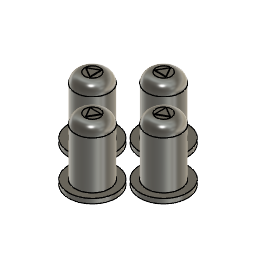
Buttons (Autodesk Fusion 360 archive; units mm, degrees)
design "D-pad"
part number: 2025-12-04-00-47-35-173
Autodesk Fusion 360 part; units mm, degrees
sketch "Sketch7" plane through (0, 0, 0) normal (0, 0, 1) x (1, 0, 0)
  circle A0 through (227.5, 10.5, -5) (220, 14.8301, -5) (220, 6.1699, -5)
  circle A1 through (226.075, 10.5, -5) (220.7125, 13.596, -5) (220.7125, 7.404, -5)
  circle A2 through (224.25, 10.5, -5) (221.625, 12.0155, -5) (221.625, 8.9845, -5)
  circle A3 through (220, 3, -5) (212.5, 7.3301, -5) (212.5, -1.3301, -5)
  circle A4 through (218.575, 3, -5) (213.2125, 6.096, -5) (213.2125, -0.096, -5)
  circle A5 through (216.75, 3, -5) (214.125, 4.5155, -5) (214.125, 1.4845, -5)
  line L0 (218, 6, -5) -> (212, 0, -5) construction
  line L1 (218, 6, -5) -> (212, 6, -5) construction
  circle A6 through (212.5, 10.5, -5) (205, 14.8301, -5) (205, 6.1699, -5)
  circle A7 through (211.075, 10.5, -5) (205.7125, 13.596, -5) (205.7125, 7.404, -5)
  circle A8 through (209.25, 10.5, -5) (206.625, 12.0155, -5) (206.625, 8.9845, -5)
  circle A9 through (218.575, 18, -5) (213.2125, 21.096, -5) (213.2125, 14.904, -5)
  circle A10 through (220, 18, -5) (212.5, 22.3301, -5) (212.5, 13.6699, -5)
  circle A11 through (216.75, 18, -5) (214.125, 19.5155, -5) (214.125, 16.4845, -5)
  point P0 (215, 3)
  dimension "d709" = 7.15
  dimension "d710" = 3.5
  dimension "d711" = 10
  dimension "d712" = 3.5
  dimension "d713" = 7.15
  dimension "d714" = 10
  dimension "d715" = 3.5
  dimension "d716" = 7.15
  dimension "d717" = 10
  dimension "d718" = 7.15
  dimension "d719" = 3.5
  dimension "d720" = 10
  dimension "d721" = 6
extrude "Extrude3" add sketch "Sketch7" along normal blind 13 contours A1 | A2 | A4 | A5 | A7 | A8 | A9 | A11 in plane through (0, 0, -5) normal (0, 0, 1) makes body 1 at (216.1386, 21.3888, 3.6667) makes body 2 at (206.3614, 7.1112, 3.6667) makes body 3 at (221.3614, 7.1112, 3.6667) makes body 4 at (216.1386, 6.3888, 3.6667)
extrude "Extrude4" add sketch "Sketch7" along normal blind 1 contours A0 | A3 | A6 | A10 in plane through (0, 0, -5) normal (0, 0, 1) bodies 1 2 3 4
extrude "Extrude5" cut sketch "Sketch7" along normal blind 6 contours A2 | A5 | A8 | A11 in plane through (0, 0, -5) normal (0, 0, 1) bodies 1 2 3 4
fillet "Fillet2" radius 2 4 faces at (216.1387, 17.6488, 8) (208.6387, 10.1488, 8) (223.6387, 10.1488, 8) (216.1387, 2.6488, 8) on bodies 1 2 3 4
sketch "Sketch9" plane through (0, 0, 8) normal (0, 0, 1) x (-1, 0, 0)
  circle A0 centre (-222.5, -10.5) radius 1.575
  line L0 (-226.5, -6.5) -> (-218.5, -6.5) construction
  line L1 (-218.5, -6.5) -> (-218.5, -14.5) construction
  line L2 (-218.5, -14.5) -> (-226.5, -14.5) construction
  line L3 (-226.5, -14.5) -> (-226.5, -6.5) construction
  line L4 (-226.5, -6.5) -> (-218.5, -14.5) construction
  line L5 (-218.5, -6.5) -> (-226.5, -14.5) construction
  line L6 (-203.5, -14.5) -> (-211.5, -14.5) construction
  line L7 (-211.5, -14.5) -> (-211.5, -6.5) construction
  line L8 (-211.5, -6.5) -> (-203.5, -6.5) construction
  line L9 (-203.5, -6.5) -> (-203.5, -14.5) construction
  line L10 (-203.5, -14.5) -> (-211.5, -6.5) construction
  line L11 (-211.5, -14.5) -> (-203.5, -6.5) construction
  line L12 (-207.5, -10.5) -> (-222.5, -10.5) construction
  line L13 (-219, 1) -> (-211, 1) construction
  line L14 (-211, 1) -> (-211, -7) construction
  line L15 (-211, -7) -> (-219, -7) construction
  line L16 (-219, -7) -> (-219, 1) construction
  line L17 (-219, 1) -> (-211, -7) construction
  line L18 (-211, 1) -> (-219, -7) construction
  line L19 (-219, -14) -> (-211, -14) construction
  line L20 (-211, -14) -> (-211, -22) construction
  line L21 (-211, -22) -> (-219, -22) construction
  line L22 (-219, -22) -> (-219, -14) construction
  line L23 (-219, -14) -> (-211, -22) construction
  line L24 (-211, -14) -> (-219, -22) construction
  line L25 (-215, -18) -> (-215, -3) construction
  line L26 (-206, -9) -> (-209, -9) construction
  line L27 (-209, -9) -> (-209, -12) construction
  line L28 (-209, -12) -> (-206, -12) construction
  line L29 (-206, -12) -> (-206, -9) construction
  line L30 (-206, -9) -> (-209, -12) construction
  line L31 (-209, -9) -> (-206, -12) construction
  line L32 (-223, -10.5) -> (-222, -10.5) construction
  line L33 (-221.796, -9.2899) -> (-223.9, -10.4954)
  line L34 (-223.9, -10.4954) -> (-221.804, -11.7147)
  line L35 (-221.804, -11.7147) -> (-221.796, -9.2899)
  line L36 (-208.2, -11.7124) -> (-206.1, -10.5)
  line L37 (-206.1, -10.5) -> (-208.2, -9.2876)
  line L38 (-208.2, -9.2876) -> (-208.2, -11.7124)
  line L39 (-221, -9) -> (-224, -9) construction
  line L40 (-224, -9) -> (-224, -12) construction
  line L41 (-224, -12) -> (-221, -12) construction
  line L42 (-221, -12) -> (-221, -9) construction
  line L43 (-221, -9) -> (-224, -12) construction
  line L44 (-224, -9) -> (-221, -12) construction
  line L45 (-216.2124, -17.3) -> (-215, -19.4)
  line L46 (-215, -19.4) -> (-213.7876, -17.3)
  line L47 (-213.7876, -17.3) -> (-216.2124, -17.3)
  line L48 (-213.7876, -3.7) -> (-215, -1.6)
  line L49 (-215, -1.6) -> (-216.2124, -3.7)
  line L50 (-216.2124, -3.7) -> (-213.7876, -3.7)
  point P0 (-222.5, -10.5)
  point P1 (-215, -3)
  point P2 (-215, -18)
  point P3 (-207.5, -10.5)
  point P4 (-222.5, -10.5)
  point P5 (-207.5, -10.5)
  point P6 (-222.5, -10.5)
  point P7 (-215, -18)
  point P8 (-215, -3)
  dimension "d731" = 8
  dimension "d732" = 8
  dimension "d735" = 8
  dimension "d736" = 8
  dimension "d737" = 8
  dimension "d738" = 8
  dimension "d739" = 8
  dimension "d740" = 8
  constraint horizontal L0
  constraint perpendicular L0 L1
  constraint parallel L0 L2
  constraint parallel L1 L3
  constraint coincident L4 P4
  constraint coincident L5 P4
  constraint coincident P4 P0
  constraint horizontal L6
  constraint vertical L7
  constraint horizontal L8
  constraint vertical L9
  constraint perpendicular L10 L11
  constraint midpoint L11 P5
  constraint horizontal L13
  constraint perpendicular L13 L14
  constraint parallel L13 L15
  constraint parallel L14 L16
  constraint coincident L17 P8
  constraint coincident L18 P8
  constraint horizontal L19
  constraint perpendicular L19 L20
  constraint parallel L19 L21
  constraint parallel L20 L22
  constraint coincident L23 P7
  constraint coincident L24 P7
  constraint coincident P7 P2
  constraint coincident P8 P1
  constraint perpendicular L15 L25
  constraint horizontal L26
  constraint perpendicular L26 L27
  constraint parallel L26 L28
  constraint parallel L27 L29
  constraint coincident L30 P5
  constraint coincident L31 P5
  constraint coincident L11 L26.start
  constraint coincident P5 P3
  constraint coincident L12 L32.end
  constraint horizontal L39
  constraint perpendicular L39 L40
  constraint parallel L39 L41
  constraint parallel L40 L42
  constraint coincident L43 P6
  constraint coincident L44 P6
  constraint coincident L5 L39.start
  constraint coincident P6 P4
  measures "d731" distance of L1.end L2.end
  measures "d732" distance of L0.end L1.end
  measures "d735" distance of L14.end L15.end
  measures "d736" distance of L13.end L14.end
  measures "d737" distance of L20.end L21.end
  measures "d738" distance of L19.end L20.end
  measures "d739" distance of L6.start L6.end
  measures "d740" distance of L6.start L8.end
extrude "Extrude7" add sketch "Sketch9" along normal blind 0.1 contours L33 L34 L35 | L36 L37 L38 | L45 L46 L47 | L48 L49 L50 bodies 1 2 3 4
fillet "Fillet3" radius 0.025 4 faces at (215, 18, 8.1) (207.5, 10.5, 8.1) (222.5, 10.5, 8.1) (215, 3, 8.1) on bodies 1 2 3 4
sketch "sketch 1269" plane through (314.9238, 31, 1.0977) normal (0, 0, 1) x (-1, 0, 0)
  circle A0 centre (99.9671, 27.0078) radius 3.6
  circle A1 centre (99.9671, 27.0078) radius 3.6
  circle A2 centre (107.4671, 19.5078) radius 3.6
  circle A3 centre (107.4671, 19.5078) radius 3.6
  circle A4 centre (99.9671, -15.4922) radius 10.5
  circle A5 centre (99.9671, -15.4922) radius 10.5
  circle A6 centre (99.9671, 12.0078) radius 3.6
  circle A7 centre (99.9671, 12.0078) radius 3.6
  circle A8 centre (92.4675, 19.584) radius 3.5995
extrude "Extrude8" cut sketch "sketch 1269" against normal blind 3 bodies 1 2 3 4
delete_face "DeleteFace1" 1 faces at (212.095, 3.0837, -1.9023) on bodies 4
delete_face "DeleteFace2" 1 faces at (204.595, 10.5837, -1.9023) on bodies 2
delete_face "DeleteFace3" 1 faces at (212.095, 18.0837, -1.9023) on bodies 1
delete_face "DeleteFace4" 1 faces at (219.5655, 10.889, -1.9023) on bodies 3

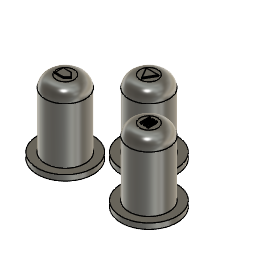
design "Menu"
part number: 2025-12-04-00-47-35-173
Autodesk Fusion 360 part; units mm, degrees
sketch "Sketch7" plane through (0, 0, 0) normal (0, 0, 1) x (1, 0, 0)
  circle A0 through (227.5, 10.5, -5) (220, 14.8301, -5) (220, 6.1699, -5)
  circle A1 through (226.075, 10.5, -5) (220.7125, 13.596, -5) (220.7125, 7.404, -5)
  circle A2 through (224.25, 10.5, -5) (221.625, 12.0155, -5) (221.625, 8.9845, -5)
  circle A3 through (220, 3, -5) (212.5, 7.3301, -5) (212.5, -1.3301, -5)
  circle A4 through (218.575, 3, -5) (213.2125, 6.096, -5) (213.2125, -0.096, -5)
  circle A5 through (216.75, 3, -5) (214.125, 4.5155, -5) (214.125, 1.4845, -5)
  line L0 (218, 6, -5) -> (212, 0, -5) construction
  line L1 (218, 6, -5) -> (212, 6, -5) construction
  circle A6 through (212.5, 10.5, -5) (205, 14.8301, -5) (205, 6.1699, -5)
  circle A7 through (211.075, 10.5, -5) (205.7125, 13.596, -5) (205.7125, 7.404, -5)
  circle A8 through (209.25, 10.5, -5) (206.625, 12.0155, -5) (206.625, 8.9845, -5)
  circle A9 through (218.575, 18, -5) (213.2125, 21.096, -5) (213.2125, 14.904, -5)
  circle A10 through (220, 18, -5) (212.5, 22.3301, -5) (212.5, 13.6699, -5)
  circle A11 through (216.75, 18, -5) (214.125, 19.5155, -5) (214.125, 16.4845, -5)
  point P0 (215, 3)
  dimension "d709" = 7.15
  dimension "d710" = 3.5
  dimension "d711" = 10
  dimension "d712" = 3.5
  dimension "d713" = 7.15
  dimension "d714" = 10
  dimension "d715" = 3.5
  dimension "d716" = 7.15
  dimension "d717" = 10
  dimension "d718" = 7.15
  dimension "d719" = 3.5
  dimension "d720" = 10
  dimension "d721" = 6
extrude "Extrude3" add sketch "Sketch7" along normal blind 13 contours A1 | A2 | A4 | A5 | A7 | A8 | A9 | A11 in plane through (0, 0, -5) normal (0, 0, 1) makes body 1 at (216.1386, 21.3888, 3.6667) makes body 2 at (206.3614, 7.1112, 3.6667) makes body 3 at (221.3614, 7.1112, 3.6667) makes body 4 at (216.1386, 6.3888, 3.6667)
extrude "Extrude4" add sketch "Sketch7" along normal blind 1 contours A0 | A3 | A6 | A10 in plane through (0, 0, -5) normal (0, 0, 1) bodies 1 2 3 4
extrude "Extrude5" cut sketch "Sketch7" along normal blind 6 contours A2 | A5 | A8 | A11 in plane through (0, 0, -5) normal (0, 0, 1) bodies 1 2 3 4
fillet "Fillet2" radius 2 4 faces at (216.1387, 17.6488, 8) (208.6387, 10.1488, 8) (223.6387, 10.1488, 8) (216.1387, 2.6488, 8) on bodies 1 2 3 4
sketch "Sketch9" plane through (0, 0, 8) normal (0, 0, 1) x (-1, 0, 0)
  circle A0 centre (-222.5, -10.5) radius 1.575
  line L0 (-226.5, -6.5) -> (-218.5, -6.5) construction
  line L1 (-218.5, -6.5) -> (-218.5, -14.5) construction
  line L2 (-218.5, -14.5) -> (-226.5, -14.5) construction
  line L3 (-226.5, -14.5) -> (-226.5, -6.5) construction
  line L4 (-226.5, -6.5) -> (-218.5, -14.5) construction
  line L5 (-218.5, -6.5) -> (-226.5, -14.5) construction
  line L6 (-203.5, -14.5) -> (-211.5, -14.5) construction
  line L7 (-211.5, -14.5) -> (-211.5, -6.5) construction
  line L8 (-211.5, -6.5) -> (-203.5, -6.5) construction
  line L9 (-203.5, -6.5) -> (-203.5, -14.5) construction
  line L10 (-203.5, -14.5) -> (-211.5, -6.5) construction
  line L11 (-211.5, -14.5) -> (-203.5, -6.5) construction
  line L12 (-207.5, -10.5) -> (-222.5, -10.5) construction
  line L13 (-219, 1) -> (-211, 1) construction
  line L14 (-211, 1) -> (-211, -7) construction
  line L15 (-211, -7) -> (-219, -7) construction
  line L16 (-219, -7) -> (-219, 1) construction
  line L17 (-219, 1) -> (-211, -7) construction
  line L18 (-211, 1) -> (-219, -7) construction
  line L19 (-219, -14) -> (-211, -14) construction
  line L20 (-211, -14) -> (-211, -22) construction
  line L21 (-211, -22) -> (-219, -22) construction
  line L22 (-219, -22) -> (-219, -14) construction
  line L23 (-219, -14) -> (-211, -22) construction
  line L24 (-211, -14) -> (-219, -22) construction
  line L25 (-215, -18) -> (-215, -3) construction
  line L26 (-206, -9) -> (-209, -9) construction
  line L27 (-209, -9) -> (-209, -12) construction
  line L28 (-209, -12) -> (-206, -12) construction
  line L29 (-206, -12) -> (-206, -9) construction
  line L30 (-206, -9) -> (-209, -12) construction
  line L31 (-209, -9) -> (-206, -12) construction
  line L32 (-223, -10.5) -> (-222, -10.5) construction
  line L33 (-221.796, -9.2899) -> (-223.9, -10.4954)
  line L34 (-223.9, -10.4954) -> (-221.804, -11.7147)
  line L35 (-221.804, -11.7147) -> (-221.796, -9.2899)
  line L36 (-208.2, -11.7124) -> (-206.1, -10.5)
  line L37 (-206.1, -10.5) -> (-208.2, -9.2876)
  line L38 (-208.2, -9.2876) -> (-208.2, -11.7124)
  line L39 (-221, -9) -> (-224, -9) construction
  line L40 (-224, -9) -> (-224, -12) construction
  line L41 (-224, -12) -> (-221, -12) construction
  line L42 (-221, -12) -> (-221, -9) construction
  line L43 (-221, -9) -> (-224, -12) construction
  line L44 (-224, -9) -> (-221, -12) construction
  line L45 (-216.2124, -17.3) -> (-215, -19.4)
  line L46 (-215, -19.4) -> (-213.7876, -17.3)
  line L47 (-213.7876, -17.3) -> (-216.2124, -17.3)
  line L48 (-213.7876, -3.7) -> (-215, -1.6)
  line L49 (-215, -1.6) -> (-216.2124, -3.7)
  line L50 (-216.2124, -3.7) -> (-213.7876, -3.7)
  point P0 (-222.5, -10.5)
  point P1 (-215, -3)
  point P2 (-215, -18)
  point P3 (-207.5, -10.5)
  point P4 (-222.5, -10.5)
  point P5 (-207.5, -10.5)
  point P6 (-222.5, -10.5)
  point P7 (-215, -18)
  point P8 (-215, -3)
  dimension "d731" = 8
  dimension "d732" = 8
  dimension "d735" = 8
  dimension "d736" = 8
  dimension "d737" = 8
  dimension "d738" = 8
  dimension "d739" = 8
  dimension "d740" = 8
  constraint horizontal L0
  constraint perpendicular L0 L1
  constraint parallel L0 L2
  constraint parallel L1 L3
  constraint coincident L4 P4
  constraint coincident L5 P4
  constraint coincident P4 P0
  constraint horizontal L6
  constraint vertical L7
  constraint horizontal L8
  constraint vertical L9
  constraint perpendicular L10 L11
  constraint midpoint L11 P5
  constraint horizontal L13
  constraint perpendicular L13 L14
  constraint parallel L13 L15
  constraint parallel L14 L16
  constraint coincident L17 P8
  constraint coincident L18 P8
  constraint horizontal L19
  constraint perpendicular L19 L20
  constraint parallel L19 L21
  constraint parallel L20 L22
  constraint coincident L23 P7
  constraint coincident L24 P7
  constraint coincident P7 P2
  constraint coincident P8 P1
  constraint perpendicular L15 L25
  constraint horizontal L26
  constraint perpendicular L26 L27
  constraint parallel L26 L28
  constraint parallel L27 L29
  constraint coincident L30 P5
  constraint coincident L31 P5
  constraint coincident L11 L26.start
  constraint coincident P5 P3
  constraint coincident L12 L32.end
  constraint horizontal L39
  constraint perpendicular L39 L40
  constraint parallel L39 L41
  constraint parallel L40 L42
  constraint coincident L43 P6
  constraint coincident L44 P6
  constraint coincident L5 L39.start
  constraint coincident P6 P4
  measures "d731" distance of L1.end L2.end
  measures "d732" distance of L0.end L1.end
  measures "d735" distance of L14.end L15.end
  measures "d736" distance of L13.end L14.end
  measures "d737" distance of L20.end L21.end
  measures "d738" distance of L19.end L20.end
  measures "d739" distance of L6.start L6.end
  measures "d740" distance of L6.start L8.end
extrude "Extrude7" add sketch "Sketch9" along normal blind 0.1 contours L33 L34 L35 | L36 L37 L38 | L45 L46 L47 | L48 L49 L50 bodies 1 2 3 4
fillet "Fillet3" radius 0.025 4 faces at (215, 18, 8.1) (207.5, 10.5, 8.1) (222.5, 10.5, 8.1) (215, 3, 8.1) on bodies 1 2 3 4
sketch "sketch 1269" plane through (314.9238, 31, 1.0977) normal (0, 0, 1) x (-1, 0, 0)
  circle A0 centre (99.9671, 27.0078) radius 3.6
  circle A1 centre (99.9671, 27.0078) radius 3.6
  circle A2 centre (107.4671, 19.5078) radius 3.6
  circle A3 centre (107.4671, 19.5078) radius 3.6
  circle A4 centre (99.9671, -15.4922) radius 10.5
  circle A5 centre (99.9671, -15.4922) radius 10.5
  circle A6 centre (99.9671, 12.0078) radius 3.6
  circle A7 centre (99.9671, 12.0078) radius 3.6
  circle A8 centre (92.4675, 19.584) radius 3.5995
extrude "Extrude8" cut sketch "sketch 1269" against normal blind 3 bodies 1 2 3 4
delete_face "DeleteFace1" 1 faces at (212.095, 3.0837, -1.9023) on bodies 4
delete_face "DeleteFace2" 1 faces at (204.595, 10.5837, -1.9023) on bodies 2
delete_face "DeleteFace3" 1 faces at (212.095, 18.0837, -1.9023) on bodies 1
delete_face "DeleteFace4" 1 faces at (219.5655, 10.889, -1.9023) on bodies 3
delete_body "RemoveBody1" bodies 4
sketch "Sketch10" plane through (0, 0, 8.1) normal (0, 0, 1) x (-1, 0, 0)
  line L0 (-221.8211, -9.3331) -> (-223.85, -10.4955)
  line L1 (-223.85, -10.4955) -> (-221.8289, -11.6714)
  line L2 (-221.8289, -11.6714) -> (-221.8211, -9.3331)
  line L3 (-216.1691, -17.325) -> (-215, -19.35)
  line L4 (-215, -19.35) -> (-213.8309, -17.325)
  line L5 (-213.8309, -17.325) -> (-216.1691, -17.325)
  line L6 (-208.175, -11.6691) -> (-206.15, -10.5)
  line L7 (-206.15, -10.5) -> (-208.175, -9.3309)
  line L8 (-208.175, -9.3309) -> (-208.175, -11.6691)
  line L9 (-205.1135, -13.6943) -> (-211.2203, -13.6943)
  line L10 (-211.2203, -13.6943) -> (-211.2203, -7.6717)
  line L11 (-211.2203, -7.6717) -> (-205.1135, -7.6717)
  line L12 (-205.1135, -7.6717) -> (-205.1135, -13.6943)
  line L13 (-212.5, -21) -> (-218.6223, -21)
  line L14 (-218.6223, -21) -> (-218.6223, -15.5953)
  line L15 (-218.6223, -15.5953) -> (-212.5, -15.5953)
  line L16 (-212.5, -15.5953) -> (-212.5, -21)
  line L17 (-219.9345, -14.3167) -> (-227, -14.3167)
  line L18 (-227, -14.3167) -> (-227, -6.5)
  line L19 (-227, -6.5) -> (-219.9345, -6.5)
  line L20 (-219.9345, -6.5) -> (-219.9345, -14.3167)
  constraint horizontal L9
  constraint vertical L10
  constraint horizontal L11
  constraint vertical L12
  constraint horizontal L13
  constraint vertical L14
  constraint horizontal L15
  constraint vertical L16
  constraint horizontal L17
  constraint vertical L18
  constraint horizontal L19
  constraint vertical L20
extrude "Extrude9" cut sketch "Sketch10" against normal up to surface (0.1 mm away) contours L0 L1 L2 | L3 L4 L5 | L6 L7 L8 | L9 L10 L11 L12 | L13 L14 L15 L16 | L17 L18 L19 L20 bodies 1 2 3
sketch "Sketch11" plane through (0, 0, 8) normal (0, 0, 1) x (-1, 0, 0)
  circle A0 centre (-207.5, -10.5) radius 1.575
  circle A1 centre (-215, -18) radius 1.575
  circle A2 centre (-222.5, -10.5) radius 1.575
  line L0 (-207.875, -11.25) -> (-206.375, -11.25)
  line L1 (-206.375, -11.25) -> (-206.375, -9.75)
  line L2 (-206.375, -9.75) -> (-207.875, -9.75)
  line L3 (-207.875, -9.75) -> (-207.875, -11.25)
  line L4 (-206.375, -10.5) -> (-208.625, -10.5) construction
  line L5 (-207.875, -11.25) -> (-208.625, -10.5)
  line L6 (-208.625, -10.5) -> (-207.875, -9.75)
  point P0 (-207.5, -10.5)
  dimension "d3" = 0.75
  dimension "d4" = 1.5
  constraint horizontal L0
  constraint vertical L1
  constraint horizontal L2
  constraint vertical L3
  constraint midpoint L1 L4.start
  constraint perpendicular L3 L4
  constraint equal L1 L2
  constraint midpoint L4 P0
  constraint coincident P0 A0.centre
  measures "d3" horizontal distance of L2.end L4.end
  measures "d4" distance of L1.end L2.end
extrude "Extrude10" add sketch "Sketch11" along normal blind 0.2 contours L0 L1 L2 L3 | L3 L5 L6 bodies 2
fillet "Fillet4" radius 0.05 5 edges at (207.125, 9.75, 8.2) (208.25, 10.125, 8.2) (208.25, 10.875, 8.2) (207.125, 11.25, 8.2) (206.375, 10.5, 8.2) on bodies 2
sketch "Sketch12" plane through (0, 0, 8) normal (0, 0, 1) x (-1, 0, 0)
  circle A0 centre (-215, -18) radius 1.575
  line L0 (-216.15, -18.664) -> (-213.85, -18.664)
  line L1 (-213.85, -18.664) -> (-215, -16.6721)
  line L2 (-215, -16.6721) -> (-216.15, -18.664)
  line L3 (-213.85, -18.664) -> (-215.575, -17.668) construction
  line L4 (-216.15, -18.664) -> (-214.425, -17.668) construction
  line L5 (-215, -16.6721) -> (-215, -18.664) construction
  point P0 (-215, -18)
  dimension "d9" = 2.3
  constraint horizontal L0
  constraint equal L0 L2
  constraint equal L0 L1
  constraint midpoint L2 L3.end
  constraint midpoint L1 L4.end
  constraint midpoint L0 L5.end
  constraint coincident L4 P0
  constraint coincident L3 P0
  constraint coincident P0 A0.centre
  measures "d9" distance of L0.start L0.end
extrude "Extrude11" add sketch "Sketch12" along normal blind 0.2 contours L0 L1 L2 bodies 1
fillet "Fillet5" radius 0.05 3 edges at (215.575, 17.668, 8.2) (215, 18.664, 8.2) (214.425, 17.668, 8.2) on bodies 1
sketch "Sketch13" plane through (0, 0, 8) normal (0, 0, 1) x (-1, 0, 0)
  circle A0 centre (-222.5, -10.5) radius 1.575
  line L0 (-223.25, -11.35) -> (-222.95, -11.35)
  line L1 (-222.95, -11.35) -> (-222.95, -9.65)
  line L2 (-222.95, -9.65) -> (-223.25, -9.65)
  line L3 (-223.25, -9.65) -> (-223.25, -11.35)
  line L4 (-222.65, -11.35) -> (-222.35, -11.35)
  line L5 (-222.35, -11.35) -> (-222.35, -9.65)
  line L6 (-222.35, -9.65) -> (-222.65, -9.65)
  line L7 (-222.65, -9.65) -> (-222.65, -11.35)
  line L8 (-222.05, -11.35) -> (-221.75, -11.35)
  line L9 (-221.75, -11.35) -> (-221.75, -9.65)
  line L10 (-221.75, -9.65) -> (-222.05, -9.65)
  line L11 (-222.05, -9.65) -> (-222.05, -11.35)
  line L12 (-222.95, -11.35) -> (-223.25, -9.65) construction
  line L13 (-223.25, -11.35) -> (-222.95, -9.65) construction
  line L14 (-222.65, -11.35) -> (-222.35, -9.65) construction
  line L15 (-222.35, -11.35) -> (-222.65, -9.65) construction
  line L16 (-222.05, -11.35) -> (-221.75, -9.65) construction
  line L17 (-222.05, -9.65) -> (-221.75, -11.35) construction
  point P0 (-223.1, -10.5)
  point P1 (-222.5, -10.5)
  point P2 (-221.9, -10.5)
  dimension "d14" = 0.3
  dimension "d15" = 0.3
  dimension "d16" = 1.7
  dimension "d17" = 0.3
  constraint horizontal L0
  constraint vertical L1
  constraint horizontal L2
  constraint vertical L3
  constraint horizontal L4
  constraint vertical L5
  constraint horizontal L6
  constraint vertical L7
  constraint horizontal L8
  constraint vertical L9
  constraint horizontal L10
  constraint vertical L11
  constraint equal L3 L7
  constraint equal L5 L11
  constraint equal L2 L6
  constraint equal L4 L8
  constraint midpoint L12 P0
  constraint midpoint L15 P1
  constraint midpoint L16 P2
  constraint horizontal P0 P1
  constraint horizontal P1 P2
  constraint coincident A0.centre P1
  measures "d14" distance of L1 L7
  measures "d15" distance of L5 L11
  measures "d16" distance of L0.start L2.end
  measures "d17" distance of L0.start L0.end
extrude "Extrude12" add sketch "Sketch13" along normal blind 0.2 contours L0 L1 L2 L3 | L4 L5 L6 L7 | L8 L9 L10 L11 bodies 3
fillet "Fillet6" radius 0.05 12 edges at (223.25, 10.5, 8.2) (223.1, 11.35, 8.2) (222.95, 10.5, 8.2) (223.1, 9.65, 8.2) (222.5, 9.65, 8.2) (222.65, 10.5, 8.2) (222.5, 11.35, 8.2) (222.35, 10.5, 8.2) (221.9, 11.35, 8.2) (222.05, 10.5, 8.2) (221.9, 9.65, 8.2) (221.75, 10.5, 8.2) on bodies 3
equation "d3 = d4 / 2"
equation "d15 = d14"
